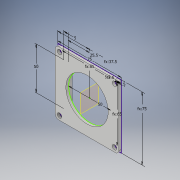
# Autodesk Inventor part: 50x5 interface
Saved by Autodesk Inventor 2019 (Build 230136000, 136)
## iProperties
Created: 2022-09-04
Part Number: 50x5 interface
Material: Generic
Document SubType Name: Modeling
Designer: laca
Density: 1 g/cm^3
Appearance: Default
Author: laca
Autodesk Inventor part; units mm, degrees
ref_plane "YZ Plane" through (0, 0, 0) normal (1, 0, 0) x (0, 1, 0)
ref_plane "XZ Plane" through (0, 0, 0) normal (0, 1, 0) x (-1, 0, 0)
ref_plane "XY Plane" through (0, 0, 0) normal (0, 0, 1) x (1, 0, 0)
sketch "Sketch1" plane through (0, 0, 0) normal (0, 0, 1) x (1, 0, 0)
  line L0 (0, 0) -> (-75, 0)
  line L1 (-75, 0) -> (-75, 75)
  line L2 (-75, 75) -> (0, 75)
  line L3 (0, 75) -> (0, 0)
  circle A0 centre (-5, 70) radius 2.65
  circle A1 centre (-70, 70) radius 2.65
  circle A2 centre (-5, 5) radius 2.65
  circle A3 centre (-70, 5) radius 2.65
  circle A4 centre (-37.5, 37.5) radius 25
  line L4 (-63, 61.5202) -> (-68, 61.5202)
  line L5 (-68, 61.5202) -> (-68, 11.5202)
  line L6 (-68, 11.5202) -> (-63, 11.5202)
  line L7 (-63, 11.5202) -> (-63, 61.5202)
  dimension "d0" = 75
  dimension "d1" = 75
  dimension "d2" = 5.3
  dimension "d3" = 5
  dimension "d4" = 5
  dimension "d7" = 65
  dimension "d10" = 65
  dimension "d26" = 50
  dimension "d29" = 50
  dimension "d30" = 5
  dimension "d31" = 25.5
  dimension "d32" = 37.5
  constraints: 16 end point, 5 centre point, 4 parallel, 3 horizontal, 2 perpendicular, 1 vertical, 6 other
  measures "d0" distance of L1.end L2.end
  measures "d1" distance of L2.end L0.start
  measures "d2" diameter of A0
  measures "d3" distance from line of L2 A0.centre
  measures "d4" distance from line of L3 A0.centre
  measures "d7" distance of A0.centre A1.centre
  measures "d10" distance of A0.centre A2.centre
  measures "d26" diameter of A4
  measures "d29" distance of L4.end L5.end
  measures "d30" distance between parallel lines of L5 L7
  measures "d31" distance from line of L7 A4.centre
  measures "d32" distance from line of L1 A4.centre
extrude "Extrusion1" add sketch "Sketch1" along normal blind 3 contours L0 L1 L2 L3 | L7 L6 L5 L4
extrude "Extrusion2" add sketch "Sketch1" against normal blind 5 contours L7 L6 L5 L4
ref_plane "Work Plane1" through (-37.5, 37.5, 0) normal (1, 0, 0) x (0, 1, 0)
mirror "Mirror1" about plane through (-37.5, 37.5, 0) normal (1, 0, 0) of "Extrusion2"
fillet "Fillet2" radius 4 2 edges at (-68, 36.5202, 0) (-7, 36.5202, 0)
fillet "Fillet3" radius 4 4 edges at (0, 0, 1.5) (-75, 0, 1.5) (-75, 75, 1.5) (0, 75, 1.5)
equation "\"d1\" = d0"
equation "\"d4\" = d3"
equation "\"d7\" = d0 - 2 * d4"
equation "\"d10\" = d1 - 2 * d3"
equation "\"d32\" = 0.5 * d0"
body "Solid1"
